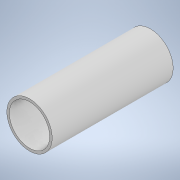
# Autodesk Inventor part: Combined_Intake_Exhaust_Manifold_2_0
Saved by Autodesk Inventor 2021 (Build 250183000, 183)
## iProperties
Created: 2021-04-23
Part Number: Combined_Intake_Exhaust_Manifold_2_0
Material: Generic
Document SubType Name: Modeling
Designer: lucia
Density: 1 g/cm^3
Appearance: Default
Author: lucia
Autodesk Inventor part; units mm, degrees
ref_plane "YZ Plane" through (0, 0, 0) normal (1, 0, 0) x (0, 1, 0)
ref_plane "XZ Plane" through (0, 0, 0) normal (0, 1, 0) x (-1, 0, 0)
ref_plane "XY Plane" through (0, 0, 0) normal (0, 0, 1) x (1, 0, 0)
sketch "Sketch1" plane through (0, 0, 0) normal (0, 0, 1) x (1, 0, 0)
  line L0 (0, 0) -> (0, -13.208)
  circle A0 centre (0, -13.208) radius 8.128
  circle A1 centre (0, -13.208) radius 12.7
  circle A2 centre (0, -13.208) radius 14.2875
  dimension "d0" = 13.208
  dimension "d1" = 16.256
  dimension "d2" = 25.4
  dimension "d3" = 28.575
  constraints: 3 centre point, 3 coincident, 2 end point, 1 vertical
  measures "d0" distance of L0.start L0.end
  measures "d1" diameter of A0
  measures "d2" diameter of A1
  measures "d3" diameter of A2
extrude "Extrusion1" add sketch "Sketch1" along normal blind 76.2 contours A2
equation "\"d0\" = 3.302 * d4"
equation "\"d1\" = 4.064 * d4"
equation "\"d2\" = 6.35 * d4"
equation "\"d5\" = 19.05 * scale"
equation "\"d4\" = 4"
equation "\"scale\" = 4"
body "Solid1"
